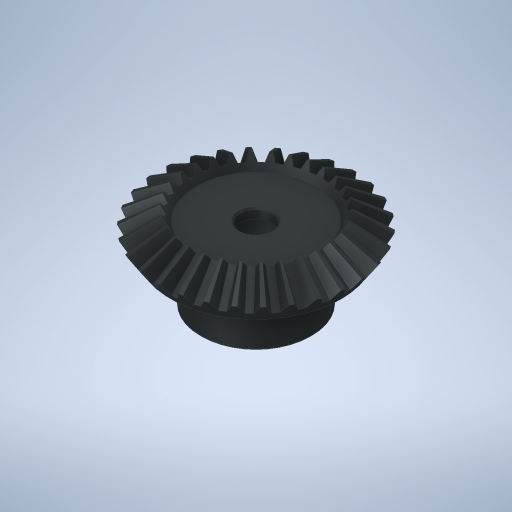
# Autodesk Inventor part: SB2-3020_On
Saved by Autodesk Inventor 2023 (Build 270158000, 158)
## iProperties
Category: PARTsolutions
Company: KHK
Created: 2023-07-20
Part Number: SB2-3020_On
Material: Iron, Cast
Catalog Web Link: www.cadenas.de
Description: Bevel Gears (SB)-R-
Vendor: KHK
Document SubType Name: Modeling
Designer: psAdmin
Manufacturer: KHK
Mass: 215.195 g
Surface Area: 104.612 cm^2
Volume: 30.0971 cm^3
Density: 7.15 g/cm^3
Appearance: Iron Gray
PSOL_IDENT_0: {$CADENAS_DATA/23d-libs/khk/bevel_gears/sb_r.prj},177 {VTYP=3D},{NB=SB2-3020_On},{LINA=SB2-3020},{NN=
PSOL_IDENT_1: Bevel Gears (SB)-R},{DATE=06.10.2022 23:14:39},{GEOMDATE=08.01.2020 09:18:20},{VERSION=},{LINEID=970
PSOL_IDENT_2: },{WBVAR=TOOTH},{WBNUMERIC=}  {NB=SB2-3020_On},{LINA=SB2-3020},{KT=DUMMY},{CN=SB2-3020},{M=2.0},{Z=3
PSOL_IDENT_3: 0},{A=10},{B=35},{C=60.0},{D=61.65},{E=40},{F=26.87},{G=21.24},{H=15.00},{I=23.0},{J=11},{K=37.56},{
PSOL_IDENT_4: L=59.27},{S=B4},{PN=SB2-2030},{WMF=B4005.WMF},{X=0.5},{Y=0.5},{R=1.0},{H1=53.33},{VERS=2},{I1=0},{I2=
PSOL_IDENT_5: 0},{AN=0},{H11=0},{TOOTH=On},{ANGLE2=0.70}
NB: SB2-3020_On
NN: Bevel Gears (SB)-R
NBSYN: $CN._$TOOTH.
LINA: SB2-3020
CATALOG: KHK
CN: SB2-3020
M: 2
Z: 30
A: 10
B: 35
C: 60
D: 61.65
E: 40
F: 26.87
G: 21.24
H: 15
I: 23
J: 11
K: 37.56
L: 59.27
S: B4
PN: SB2-2030
WMF: B4005.WMF
X: 0.5
Y: 0.5
R: 1
H1: 53.33
VERS: 2
I1: 0
I2: 0
AN: 0
H11: 0
TOOTH: On
ANGLE2: 0.7
SUPPLIER: KHK
ARTICLENO: SB2-3020_On
BOMINFO: SB2-3020
CREATOR: CADENAS GmbH
Title: SB2-3020
Author: Cadenas PARTsolutions
Autodesk Inventor part; units mm, degrees
ref_plane "YZ Plane" through (0, 0, 0) normal (1, 0, 0) x (0, 1, 0)
ref_plane "XZ Plane" through (0, 0, 0) normal (0, 1, 0) x (-1, 0, 0)
ref_plane "XY Plane" through (0, 0, 0) normal (0, 0, 1) x (1, 0, 0)
sketch "Sketch_14" plane through (0, -13.13, 0) normal (0, -1, 0) x (1, 0, 0)
  arc A0 (0.2734, -21.7526) -> (1.13, -15.3877) centre (-116.736, -2.7646) ccw
  arc A1 (1.13, -15.3877) -> (2.094, -15.2863) centre (0, 0) ccw
  arc A2 (2.094, -15.2863) -> (4.2552, -21.3341) centre (114.7598, 21.5666) ccw
  arc A3 (4.2552, -21.3341) -> (4.79, -21.2204) centre (0, 0) ccw
  arc A4 (4.79, -21.2204) -> (4.3046, -14.8165) centre (-113.6102, -26.975) ccw
  arc A5 (4.3046, -14.8165) -> (5.2264, -14.5169) centre (0, 0) ccw
  arc A6 (5.2264, -14.5169) -> (8.5978, -19.9832) centre (107.7681, 44.9552) ccw
  arc A7 (8.5978, -19.9832) -> (9.0973, -19.7608) centre (0, 0) ccw
  arc A8 (9.0973, -19.7608) -> (7.291, -13.5977) centre (-105.5192, -50.0064) ccw
  arc A9 (7.291, -13.5977) -> (8.1304, -13.1131) centre (0, 0) ccw
  arc A10 (8.1304, -13.1131) -> (12.5647, -17.7589) centre (96.0664, 66.3791) ccw
  arc A11 (12.5647, -17.7589) -> (13.007, -17.4375) centre (0, 0) ccw
  arc A12 (13.007, -17.4375) -> (9.9588, -11.7847) centre (-92.8164, -70.8523) ccw
  arc A13 (9.9588, -11.7847) -> (10.6791, -11.1361) centre (0, 0) ccw
  arc A14 (10.6791, -11.1361) -> (15.9824, -14.7585) centre (80.1661, 84.9019) ccw
  arc A15 (15.9824, -14.7585) -> (16.3482, -14.3522) centre (0, 0) ccw
  arc A16 (16.3482, -14.3522) -> (12.1914, -9.4566) centre (-76.0571, -88.6016) ccw
  arc A17 (12.1914, -9.4566) -> (12.7611, -8.6724) centre (0, 0) ccw
  arc A18 (12.7611, -8.6724) -> (18.7016, -11.113) centre (60.7622, 99.714) ccw
  arc A19 (18.7016, -11.113) -> (18.975, -10.6395) centre (0, 0) ccw
  arc A20 (18.975, -10.6395) -> (13.8911, -6.7152) centre (-55.9738, -102.4786) ccw
  arc A21 (13.8911, -6.7152) -> (14.2853, -5.8297) centre (0, 0) ccw
  arc A22 (14.2853, -5.8297) -> (20.6035, -6.9819) centre (38.7027, 110.1682) ccw
  arc A23 (20.6035, -6.9819) -> (20.7724, -6.4619) centre (0, 0) ccw
  arc A24 (20.7724, -6.4619) -> (14.9837, -3.6804) centre (-33.4441, -111.8768) ccw
  arc A25 (14.9837, -3.6804) -> (15.1852, -2.7323) centre (0, 0) ccw
  arc A26 (15.1852, -2.7323) -> (21.6048, -2.5456) centre (14.9517, 115.8075) ccw
  arc A27 (21.6048, -2.5456) -> (21.662, -2.0019) centre (0, 0) ccw
  arc A28 (21.662, -2.0019) -> (15.4215, -0.4846) centre (-9.4528, -116.3855) ccw
  arc A29 (15.4215, -0.4846) -> (15.4215, 0.4846) centre (0, 0) ccw
  arc A30 (15.4215, 0.4846) -> (21.662, 2.0019) centre (-9.4528, 116.3855) ccw
  arc A31 (21.662, 2.0019) -> (21.6048, 2.5456) centre (0, 0) ccw
  arc A32 (21.6048, 2.5456) -> (15.1852, 2.7323) centre (14.9517, -115.8075) ccw
  arc A33 (15.1852, 2.7323) -> (14.9837, 3.6804) centre (0, 0) ccw
  arc A34 (14.9837, 3.6804) -> (20.7724, 6.4619) centre (-33.4441, 111.8768) ccw
  arc A35 (20.7724, 6.4619) -> (20.6035, 6.9819) centre (0, 0) ccw
  arc A36 (20.6035, 6.9819) -> (14.2853, 5.8297) centre (38.7027, -110.1682) ccw
  arc A37 (14.2853, 5.8297) -> (13.8911, 6.7152) centre (0, 0) ccw
  arc A38 (13.8911, 6.7152) -> (18.975, 10.6395) centre (-55.9738, 102.4786) ccw
  arc A39 (18.975, 10.6395) -> (18.7016, 11.113) centre (0, 0) ccw
  arc A40 (18.7016, 11.113) -> (12.7611, 8.6724) centre (60.7622, -99.714) ccw
  arc A41 (12.7611, 8.6724) -> (12.1914, 9.4566) centre (0, 0) ccw
  arc A42 (12.1914, 9.4566) -> (16.3482, 14.3522) centre (-76.0571, 88.6016) ccw
  arc A43 (16.3482, 14.3522) -> (15.9824, 14.7585) centre (0, 0) ccw
  arc A44 (15.9824, 14.7585) -> (10.6791, 11.1361) centre (80.1661, -84.9019) ccw
  arc A45 (10.6791, 11.1361) -> (9.9588, 11.7847) centre (0, 0) ccw
  arc A46 (9.9588, 11.7847) -> (13.007, 17.4375) centre (-92.8164, 70.8523) ccw
  arc A47 (13.007, 17.4375) -> (12.5647, 17.7589) centre (0, 0) ccw
  arc A48 (12.5647, 17.7589) -> (8.1304, 13.1131) centre (96.0664, -66.3791) ccw
  arc A49 (8.1304, 13.1131) -> (7.291, 13.5977) centre (0, 0) ccw
  arc A50 (7.291, 13.5977) -> (9.0973, 19.7608) centre (-105.5192, 50.0064) ccw
  arc A51 (9.0973, 19.7608) -> (8.5978, 19.9832) centre (0, 0) ccw
  arc A52 (8.5978, 19.9832) -> (5.2264, 14.5169) centre (107.7681, -44.9552) ccw
  arc A53 (5.2264, 14.5169) -> (4.3046, 14.8165) centre (0, 0) ccw
  arc A54 (4.3046, 14.8165) -> (4.79, 21.2204) centre (-113.6102, 26.975) ccw
  arc A55 (4.79, 21.2204) -> (4.2552, 21.3341) centre (0, 0) ccw
  arc A56 (4.2552, 21.3341) -> (2.094, 15.2863) centre (114.7598, -21.5666) ccw
  arc A57 (2.094, 15.2863) -> (1.13, 15.3877) centre (0, 0) ccw
  arc A58 (1.13, 15.3877) -> (0.2734, 21.7526) centre (-116.736, 2.7646) ccw
  arc A59 (0.2734, 21.7526) -> (-0.2734, 21.7526) centre (0, 0) ccw
  arc A60 (-0.2734, 21.7526) -> (-1.13, 15.3877) centre (116.736, 2.7646) ccw
  arc A61 (-1.13, 15.3877) -> (-2.094, 15.2863) centre (0, 0) ccw
  arc A62 (-2.094, 15.2863) -> (-4.2552, 21.3341) centre (-114.7598, -21.5666) ccw
  arc A63 (-4.2552, 21.3341) -> (-4.79, 21.2204) centre (0, 0) ccw
  arc A64 (-4.79, 21.2204) -> (-4.3046, 14.8165) centre (113.6102, 26.975) ccw
  arc A65 (-4.3046, 14.8165) -> (-5.2264, 14.5169) centre (0, 0) ccw
  arc A66 (-5.2264, 14.5169) -> (-8.5978, 19.9832) centre (-107.7681, -44.9552) ccw
  arc A67 (-8.5978, 19.9832) -> (-9.0973, 19.7608) centre (0, 0) ccw
  arc A68 (-9.0973, 19.7608) -> (-7.291, 13.5977) centre (105.5192, 50.0064) ccw
  arc A69 (-7.291, 13.5977) -> (-8.1304, 13.1131) centre (0, 0) ccw
  arc A70 (-8.1304, 13.1131) -> (-12.5647, 17.7589) centre (-96.0664, -66.3791) ccw
  arc A71 (-12.5647, 17.7589) -> (-13.007, 17.4375) centre (0, 0) ccw
  arc A72 (-13.007, 17.4375) -> (-9.9588, 11.7847) centre (92.8164, 70.8523) ccw
  arc A73 (-9.9588, 11.7847) -> (-10.6791, 11.1361) centre (0, 0) ccw
  arc A74 (-10.6791, 11.1361) -> (-15.9824, 14.7585) centre (-80.1661, -84.9019) ccw
  arc A75 (-15.9824, 14.7585) -> (-16.3482, 14.3522) centre (0, 0) ccw
  arc A76 (-16.3482, 14.3522) -> (-12.1914, 9.4566) centre (76.0571, 88.6016) ccw
  arc A77 (-12.1914, 9.4566) -> (-12.7611, 8.6724) centre (0, 0) ccw
  arc A78 (-12.7611, 8.6724) -> (-18.7016, 11.113) centre (-60.7622, -99.714) ccw
  arc A79 (-18.7016, 11.113) -> (-18.975, 10.6395) centre (0, 0) ccw
  arc A80 (-18.975, 10.6395) -> (-13.8911, 6.7152) centre (55.9738, 102.4786) ccw
  arc A81 (-13.8911, 6.7152) -> (-14.2853, 5.8297) centre (0, 0) ccw
  arc A82 (-14.2853, 5.8297) -> (-20.6035, 6.9819) centre (-38.7027, -110.1682) ccw
  arc A83 (-20.6035, 6.9819) -> (-20.7724, 6.4619) centre (0, 0) ccw
  arc A84 (-20.7724, 6.4619) -> (-14.9837, 3.6804) centre (33.4441, 111.8768) ccw
  arc A85 (-14.9837, 3.6804) -> (-15.1852, 2.7323) centre (0, 0) ccw
  arc A86 (-15.1852, 2.7323) -> (-21.6048, 2.5456) centre (-14.9517, -115.8075) ccw
  arc A87 (-21.6048, 2.5456) -> (-21.662, 2.0019) centre (0, 0) ccw
  arc A88 (-21.662, 2.0019) -> (-15.4215, 0.4846) centre (9.4528, 116.3855) ccw
  arc A89 (-15.4215, 0.4846) -> (-15.4215, -0.4846) centre (0, 0) ccw
  arc A90 (-15.4215, -0.4846) -> (-21.662, -2.0019) centre (9.4528, -116.3855) ccw
  arc A91 (-21.662, -2.0019) -> (-21.6048, -2.5456) centre (0, 0) ccw
  arc A92 (-21.6048, -2.5456) -> (-15.1852, -2.7323) centre (-14.9517, 115.8075) ccw
  arc A93 (-15.1852, -2.7323) -> (-14.9837, -3.6804) centre (0, 0) ccw
  arc A94 (-14.9837, -3.6804) -> (-20.7724, -6.4619) centre (33.4441, -111.8768) ccw
  arc A95 (-20.7724, -6.4619) -> (-20.6035, -6.9819) centre (0, 0) ccw
  arc A96 (-20.6035, -6.9819) -> (-14.2853, -5.8297) centre (-38.7027, 110.1682) ccw
  arc A97 (-14.2853, -5.8297) -> (-13.8911, -6.7152) centre (0, 0) ccw
  arc A98 (-13.8911, -6.7152) -> (-18.975, -10.6395) centre (55.9738, -102.4786) ccw
  arc A99 (-18.975, -10.6395) -> (-18.7016, -11.113) centre (0, 0) ccw
  arc A100 (-18.7016, -11.113) -> (-12.7611, -8.6724) centre (-60.7622, 99.714) ccw
  arc A101 (-12.7611, -8.6724) -> (-12.1914, -9.4566) centre (0, 0) ccw
  arc A102 (-12.1914, -9.4566) -> (-16.3482, -14.3522) centre (76.0571, -88.6016) ccw
  arc A103 (-16.3482, -14.3522) -> (-15.9824, -14.7585) centre (0, 0) ccw
  arc A104 (-15.9824, -14.7585) -> (-10.6791, -11.1361) centre (-80.1661, 84.9019) ccw
  arc A105 (-10.6791, -11.1361) -> (-9.9588, -11.7847) centre (0, 0) ccw
  arc A106 (-9.9588, -11.7847) -> (-13.007, -17.4375) centre (92.8164, -70.8523) ccw
  arc A107 (-13.007, -17.4375) -> (-12.5647, -17.7589) centre (0, 0) ccw
  arc A108 (-12.5647, -17.7589) -> (-8.1304, -13.1131) centre (-96.0664, 66.3791) ccw
  arc A109 (-8.1304, -13.1131) -> (-7.291, -13.5977) centre (0, 0) ccw
  arc A110 (-7.291, -13.5977) -> (-9.0973, -19.7608) centre (105.5192, -50.0064) ccw
  arc A111 (-9.0973, -19.7608) -> (-8.5978, -19.9832) centre (0, 0) ccw
  arc A112 (-8.5978, -19.9832) -> (-5.2264, -14.5169) centre (-107.7681, 44.9552) ccw
  arc A113 (-5.2264, -14.5169) -> (-4.3046, -14.8165) centre (0, 0) ccw
  arc A114 (-4.3046, -14.8165) -> (-4.79, -21.2204) centre (113.6102, -26.975) ccw
  arc A115 (-4.79, -21.2204) -> (-4.2552, -21.3341) centre (0, 0) ccw
  arc A116 (-4.2552, -21.3341) -> (-2.094, -15.2863) centre (-114.7598, 21.5666) ccw
  arc A117 (-2.094, -15.2863) -> (-1.13, -15.3877) centre (0, 0) ccw
  arc A118 (-1.13, -15.3877) -> (-0.2734, -21.7526) centre (116.736, -2.7646) ccw
  arc A119 (-0.2734, -21.7526) -> (0.2734, -21.7526) centre (0, 0) ccw
  constraints: 240 point on circle, 120 centre point
sketch "Sketch_15" plane through (0, -25, 0) normal (0, -1, 0) x (1, 0, 0)
  arc A0 (0.55, -43.7655) -> (2.4237, -33.0051) centre (-290.4201, 12.4458) ccw
  arc A1 (2.4237, -33.0051) -> (4.4914, -32.7878) centre (0, 0) ccw
  arc A2 (4.4914, -32.7878) -> (8.5614, -42.9234) centre (281.4861, 72.5555) ccw
  arc A3 (8.5614, -42.9234) -> (9.6373, -42.6947) centre (0, 0) ccw
  arc A4 (9.6373, -42.6947) -> (9.2329, -31.78) centre (-286.6614, -48.208) ccw
  arc A5 (9.2329, -31.78) -> (11.2102, -31.1375) centre (0, 0) ccw
  arc A6 (11.2102, -31.1375) -> (17.2986, -40.2055) centre (260.2499, 129.4943) ccw
  arc A7 (17.2986, -40.2055) -> (18.3035, -39.758) centre (0, 0) ccw
  arc A8 (18.3035, -39.758) -> (15.6386, -29.1659) centre (-270.3741, -106.7547) ccw
  arc A9 (15.6386, -29.1659) -> (17.4391, -28.1264) centre (0, 0) ccw
  arc A10 (17.4391, -28.1264) -> (25.2797, -35.7303) centre (227.6394, 180.7735) ccw
  arc A11 (25.2797, -35.7303) -> (26.1697, -35.0837) centre (0, 0) ccw
  arc A12 (26.1697, -35.0837) -> (21.3608, -25.2771) centre (-242.2703, -160.6358) ccw
  arc A13 (21.3608, -25.2771) -> (22.9058, -23.8859) centre (0, 0) ccw
  arc A14 (22.9058, -23.8859) -> (32.1561, -29.6935) centre (185.08, 224.1521) ccw
  arc A15 (32.1561, -29.6935) -> (32.8921, -28.8761) centre (0, 0) ccw
  arc A16 (32.8921, -28.8761) -> (26.1494, -20.2836) centre (-203.578, -207.4964) ccw
  arc A17 (26.1494, -20.2836) -> (27.3714, -18.6016) centre (0, 0) ccw
  arc A18 (27.3714, -18.6016) -> (37.627, -22.3591) centre (134.4317, 257.7341) ccw
  arc A19 (37.627, -22.3591) -> (38.177, -21.4064) centre (0, 0) ccw
  arc A20 (38.177, -21.4064) -> (29.7952, -14.4035) centre (-155.9884, -245.2883) ccw
  arc A21 (29.7952, -14.4035) -> (30.6408, -12.5043) centre (0, 0) ccw
  arc A22 (30.6408, -12.5043) -> (41.4535, -14.0474) centre (77.9081, 280.0519) ccw
  arc A23 (41.4535, -14.0474) -> (41.7934, -13.0012) centre (0, 0) ccw
  arc A24 (41.7934, -13.0012) -> (32.1387, -7.894) centre (-101.5814, -272.36) ccw
  arc A25 (32.1387, -7.894) -> (32.571, -5.8604) centre (0, 0) ccw
  arc A26 (32.571, -5.8604) -> (43.4682, -5.1217) centre (17.9796, 290.1301) ccw
  arc A27 (43.4682, -5.1217) -> (43.5832, -4.0277) centre (0, 0) ccw
  arc A28 (43.5832, -4.0277) -> (33.0777, -1.0395) centre (-42.7347, -287.5282) ccw
  arc A29 (33.0777, -1.0395) -> (33.0777, 1.0395) centre (0, 0) ccw
  arc A30 (33.0777, 1.0395) -> (43.5832, 4.0277) centre (-42.7347, 287.5282) ccw
  arc A31 (43.5832, 4.0277) -> (43.4682, 5.1217) centre (0, 0) ccw
  arc A32 (43.4682, 5.1217) -> (32.571, 5.8604) centre (17.9796, -290.1301) ccw
  arc A33 (32.571, 5.8604) -> (32.1387, 7.894) centre (0, 0) ccw
  arc A34 (32.1387, 7.894) -> (41.7934, 13.0012) centre (-101.5814, 272.36) ccw
  arc A35 (41.7934, 13.0012) -> (41.4535, 14.0474) centre (0, 0) ccw
  arc A36 (41.4535, 14.0474) -> (30.6408, 12.5043) centre (77.9081, -280.0519) ccw
  arc A37 (30.6408, 12.5043) -> (29.7952, 14.4035) centre (0, 0) ccw
  arc A38 (29.7952, 14.4035) -> (38.177, 21.4064) centre (-155.9884, 245.2883) ccw
  arc A39 (38.177, 21.4064) -> (37.627, 22.3591) centre (0, 0) ccw
  arc A40 (37.627, 22.3591) -> (27.3714, 18.6016) centre (134.4317, -257.7341) ccw
  arc A41 (27.3714, 18.6016) -> (26.1494, 20.2836) centre (0, 0) ccw
  arc A42 (26.1494, 20.2836) -> (32.8921, 28.8761) centre (-203.578, 207.4964) ccw
  arc A43 (32.8921, 28.8761) -> (32.1561, 29.6935) centre (0, 0) ccw
  arc A44 (32.1561, 29.6935) -> (22.9058, 23.8859) centre (185.08, -224.1521) ccw
  arc A45 (22.9058, 23.8859) -> (21.3608, 25.2771) centre (0, 0) ccw
  arc A46 (21.3608, 25.2771) -> (26.1697, 35.0837) centre (-242.2703, 160.6358) ccw
  arc A47 (26.1697, 35.0837) -> (25.2797, 35.7303) centre (0, 0) ccw
  arc A48 (25.2797, 35.7303) -> (17.4391, 28.1264) centre (227.6394, -180.7735) ccw
  arc A49 (17.4391, 28.1264) -> (15.6386, 29.1659) centre (0, 0) ccw
  arc A50 (15.6386, 29.1659) -> (18.3035, 39.758) centre (-270.3741, 106.7547) ccw
  arc A51 (18.3035, 39.758) -> (17.2986, 40.2055) centre (0, 0) ccw
  arc A52 (17.2986, 40.2055) -> (11.2102, 31.1375) centre (260.2499, -129.4943) ccw
  arc A53 (11.2102, 31.1375) -> (9.2329, 31.78) centre (0, 0) ccw
  arc A54 (9.2329, 31.78) -> (9.6373, 42.6947) centre (-286.6614, 48.208) ccw
  arc A55 (9.6373, 42.6947) -> (8.5614, 42.9234) centre (0, 0) ccw
  arc A56 (8.5614, 42.9234) -> (4.4914, 32.7878) centre (281.4861, -72.5555) ccw
  arc A57 (4.4914, 32.7878) -> (2.4237, 33.0051) centre (0, 0) ccw
  arc A58 (2.4237, 33.0051) -> (0.55, 43.7655) centre (-290.4201, -12.4458) ccw
  arc A59 (0.55, 43.7655) -> (-0.55, 43.7655) centre (0, 0) ccw
  arc A60 (-0.55, 43.7655) -> (-2.4237, 33.0051) centre (290.4201, -12.4458) ccw
  arc A61 (-2.4237, 33.0051) -> (-4.4914, 32.7878) centre (0, 0) ccw
  arc A62 (-4.4914, 32.7878) -> (-8.5614, 42.9234) centre (-281.4861, -72.5555) ccw
  arc A63 (-8.5614, 42.9234) -> (-9.6373, 42.6947) centre (0, 0) ccw
  arc A64 (-9.6373, 42.6947) -> (-9.2329, 31.78) centre (286.6614, 48.208) ccw
  arc A65 (-9.2329, 31.78) -> (-11.2102, 31.1375) centre (0, 0) ccw
  arc A66 (-11.2102, 31.1375) -> (-17.2986, 40.2055) centre (-260.2499, -129.4943) ccw
  arc A67 (-17.2986, 40.2055) -> (-18.3035, 39.758) centre (0, 0) ccw
  arc A68 (-18.3035, 39.758) -> (-15.6386, 29.1659) centre (270.3741, 106.7547) ccw
  arc A69 (-15.6386, 29.1659) -> (-17.4391, 28.1264) centre (0, 0) ccw
  arc A70 (-17.4391, 28.1264) -> (-25.2797, 35.7303) centre (-227.6394, -180.7735) ccw
  arc A71 (-25.2797, 35.7303) -> (-26.1697, 35.0837) centre (0, 0) ccw
  arc A72 (-26.1697, 35.0837) -> (-21.3608, 25.2771) centre (242.2703, 160.6358) ccw
  arc A73 (-21.3608, 25.2771) -> (-22.9058, 23.8859) centre (0, 0) ccw
  arc A74 (-22.9058, 23.8859) -> (-32.1561, 29.6935) centre (-185.08, -224.1521) ccw
  arc A75 (-32.1561, 29.6935) -> (-32.8921, 28.8761) centre (0, 0) ccw
  arc A76 (-32.8921, 28.8761) -> (-26.1494, 20.2836) centre (203.578, 207.4964) ccw
  arc A77 (-26.1494, 20.2836) -> (-27.3714, 18.6016) centre (0, 0) ccw
  arc A78 (-27.3714, 18.6016) -> (-37.627, 22.3591) centre (-134.4317, -257.7341) ccw
  arc A79 (-37.627, 22.3591) -> (-38.177, 21.4064) centre (0, 0) ccw
  arc A80 (-38.177, 21.4064) -> (-29.7952, 14.4035) centre (155.9884, 245.2883) ccw
  arc A81 (-29.7952, 14.4035) -> (-30.6408, 12.5043) centre (0, 0) ccw
  arc A82 (-30.6408, 12.5043) -> (-41.4535, 14.0474) centre (-77.9081, -280.0519) ccw
  arc A83 (-41.4535, 14.0474) -> (-41.7934, 13.0012) centre (0, 0) ccw
  arc A84 (-41.7934, 13.0012) -> (-32.1387, 7.894) centre (101.5814, 272.36) ccw
  arc A85 (-32.1387, 7.894) -> (-32.571, 5.8604) centre (0, 0) ccw
  arc A86 (-32.571, 5.8604) -> (-43.4682, 5.1217) centre (-17.9796, -290.1301) ccw
  arc A87 (-43.4682, 5.1217) -> (-43.5832, 4.0277) centre (0, 0) ccw
  arc A88 (-43.5832, 4.0277) -> (-33.0777, 1.0395) centre (42.7347, 287.5282) ccw
  arc A89 (-33.0777, 1.0395) -> (-33.0777, -1.0395) centre (0, 0) ccw
  arc A90 (-33.0777, -1.0395) -> (-43.5832, -4.0277) centre (42.7347, -287.5282) ccw
  arc A91 (-43.5832, -4.0277) -> (-43.4682, -5.1217) centre (0, 0) ccw
  arc A92 (-43.4682, -5.1217) -> (-32.571, -5.8604) centre (-17.9796, 290.1301) ccw
  arc A93 (-32.571, -5.8604) -> (-32.1387, -7.894) centre (0, 0) ccw
  arc A94 (-32.1387, -7.894) -> (-41.7934, -13.0012) centre (101.5814, -272.36) ccw
  arc A95 (-41.7934, -13.0012) -> (-41.4535, -14.0474) centre (0, 0) ccw
  arc A96 (-41.4535, -14.0474) -> (-30.6408, -12.5043) centre (-77.9081, 280.0519) ccw
  arc A97 (-30.6408, -12.5043) -> (-29.7952, -14.4035) centre (0, 0) ccw
  arc A98 (-29.7952, -14.4035) -> (-38.177, -21.4064) centre (155.9884, -245.2883) ccw
  arc A99 (-38.177, -21.4064) -> (-37.627, -22.3591) centre (0, 0) ccw
  arc A100 (-37.627, -22.3591) -> (-27.3714, -18.6016) centre (-134.4317, 257.7341) ccw
  arc A101 (-27.3714, -18.6016) -> (-26.1494, -20.2836) centre (0, 0) ccw
  arc A102 (-26.1494, -20.2836) -> (-32.8921, -28.8761) centre (203.578, -207.4964) ccw
  arc A103 (-32.8921, -28.8761) -> (-32.1561, -29.6935) centre (0, 0) ccw
  arc A104 (-32.1561, -29.6935) -> (-22.9058, -23.8859) centre (-185.08, 224.1521) ccw
  arc A105 (-22.9058, -23.8859) -> (-21.3608, -25.2771) centre (0, 0) ccw
  arc A106 (-21.3608, -25.2771) -> (-26.1697, -35.0837) centre (242.2703, -160.6358) ccw
  arc A107 (-26.1697, -35.0837) -> (-25.2797, -35.7303) centre (0, 0) ccw
  arc A108 (-25.2797, -35.7303) -> (-17.4391, -28.1264) centre (-227.6394, 180.7735) ccw
  arc A109 (-17.4391, -28.1264) -> (-15.6386, -29.1659) centre (0, 0) ccw
  arc A110 (-15.6386, -29.1659) -> (-18.3035, -39.758) centre (270.3741, -106.7547) ccw
  arc A111 (-18.3035, -39.758) -> (-17.2986, -40.2055) centre (0, 0) ccw
  arc A112 (-17.2986, -40.2055) -> (-11.2102, -31.1375) centre (-260.2499, 129.4943) ccw
  arc A113 (-11.2102, -31.1375) -> (-9.2329, -31.78) centre (0, 0) ccw
  arc A114 (-9.2329, -31.78) -> (-9.6373, -42.6947) centre (286.6614, -48.208) ccw
  arc A115 (-9.6373, -42.6947) -> (-8.5614, -42.9234) centre (0, 0) ccw
  arc A116 (-8.5614, -42.9234) -> (-4.4914, -32.7878) centre (-281.4861, 72.5555) ccw
  arc A117 (-4.4914, -32.7878) -> (-2.4237, -33.0051) centre (0, 0) ccw
  arc A118 (-2.4237, -33.0051) -> (-0.55, -43.7655) centre (290.4201, 12.4458) ccw
  arc A119 (-0.55, -43.7655) -> (0.55, -43.7655) centre (0, 0) ccw
  constraints: 240 point on circle, 120 centre point
loft "Loft1" add profiles "Sketch_14", "Sketch_15"
sketch "Sketch_9" plane through (0, 0, 0) normal (0, 0, 1) x (1, 0, 0)
  line L0 (0, -13.13) -> (0, -40)
  line L1 (0, -40) -> (-17, -40)
  line L2 (-17, -40) -> (-17.5, -39.5)
  line L3 (-17.5, -39.5) -> (-17.5, -26)
  arc A0 (-17.5, -26) -> (-18.5, -25) centre (-18.5, -26) ccw
  line L4 (-18.5, -25) -> (-26.665, -25)
  line L5 (-26.665, -25) -> (-28.6846, -21.9705)
  line L6 (-28.6846, -21.9705) -> (-19.9942, -15.1702)
  line L7 (-19.9942, -15.1702) -> (-18.7743, -17)
  line L8 (-18.7743, -17) -> (0, -17)
  line L9 (0, -17) -> (0, -40)
  constraints: 20 end point, 2 point on circle, 1 centre point
revolve "Revolution1" add sketch "Sketch_9" angle 360 about axis through (0, -13.13, 0) along (0, 1, 0)
sketch "Sketch_10" plane through (0, 0, 0) normal (0, 0, 1) x (1, 0, 0)
  line L0 (0, 0) -> (0, -40)
  line L1 (0, -40) -> (-5.5, -40)
  line L2 (-5.5, -40) -> (-5, -39.5)
  line L3 (-5, -39.5) -> (-5, -17.5)
  line L4 (-5, -17.5) -> (-5.5, -17)
  line L5 (-5.5, -17) -> (-18.7743, -17)
  line L6 (-18.7743, -17) -> (-21.3543, -13.13)
  line L7 (-21.3543, -13.13) -> (-30.825, -18.76)
  line L8 (-30.825, -18.76) -> (-26.665, -25)
  line L9 (-26.665, -25) -> (-73.98, -25)
  line L10 (-73.98, -25) -> (-73.98, 0)
  line L11 (-73.98, 0) -> (0, 0)
  line L12 (0, 0) -> (0, -40)
  constraints: 26 end point
revolve "Revolution2" cut sketch "Sketch_10" angle 360 about axis through (0, 0, 0) along (0, 1, 0)
ref_plane "IP2_XY" through (0, 0, 0) normal (0, 0, 1) x (1, 0, 0)
ref_plane "IP2_YZ" through (0, 0, 0) normal (1, 0, 0) x (0, 1, 0)
ref_plane "IP2_ZX" through (0, 0, 0) normal (0, 1, 0) x (0, 0, 1)
ref_plane "dummy_XY" through (0, 0, 0) normal (0, 1, 0) x (1, 0, 0)
ref_plane "dummy_YZ" through (0, 0, 0) normal (1, 0, 0) x (0, 0, -1)
ref_plane "dummy_ZX" through (0, 0, 0) normal (0, 0, -1) x (0, 1, 0)
ref_plane "r_XY" through (0, 0, 0) normal (0, 1, 0) x (1, 0, 0)
ref_plane "r_YZ" through (0, 0, 0) normal (1, 0, 0) x (0, 0, -1)
ref_plane "r_ZX" through (0, 0, 0) normal (0, 0, -1) x (0, 1, 0)
sketch "Sketch5" plane through (0, -40, 0) normal (0, -1, 0) x (1, 0, 0)
  circle A0 centre (0, 0) radius 8
  line L0 (10.5, 2.5) -> (5.5, 2.5)
  line L1 (5.5, 2.5) -> (5.5, -2.5)
  line L2 (5.5, -2.5) -> (10.5, -2.5)
  line L3 (10.5, -2.5) -> (10.5, 2.5)
  line L4 (10.5, 2.5) -> (5.5, -2.5) construction
  line L5 (5.5, 2.5) -> (10.5, -2.5) construction
  point P0 (8, 0)
  point P1 (7.5993, 2.5)
  point P2 (7.5993, -2.5)
  dimension "d8" = 16
  dimension "d6" = 5
  dimension "d7" = 2.5
  constraints: 12 end point, 2 midpoint, 2 parallel, 1 coincident, 1 horizontal, 1 horizontal alignment, 1 perpendicular, 3 other
  measures "d6" distance of L2.end L0.start
  measures "d7" distance from line of point (8, 0) L3
extrude "Extrusion1" cut sketch "Sketch5" against normal blind 20
body "Solid1"
